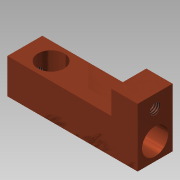
# Autodesk Inventor part: Part26
Saved by Autodesk Inventor 2014 (Build 180170000, 170)
## iProperties
Created: 2015-09-27
Part Number: Part26
Material: Copper
Document SubType Name: Modeling
Designer: Administrator
Density: 1 g/cm^3
Appearance: Copper - Satin
Author: Administrator
Autodesk Inventor part; units mm, degrees
ref_plane "YZ Plane" through (0, 0, 0) normal (1, 0, 0) x (0, 1, 0)
ref_plane "XZ Plane" through (0, 0, 0) normal (0, 1, 0) x (-1, 0, 0)
ref_plane "XY Plane" through (0, 0, 0) normal (0, 0, 1) x (1, 0, 0)
sketch "Sketch1" plane through (0, 0, 0) normal (0, 0, 1) x (1, 0, 0)
  circle A0 centre (0, 0) radius 3 projected
  line L0 (6, -4) -> (-6, -4)
  line L1 (-6, -4) -> (-6, 4)
  line L2 (-6, 4) -> (6, 4)
  line L3 (6, 4) -> (6, -4)
  line L4 (6, -4) -> (-6, 4) construction
  line L5 (-6, -4) -> (6, 4) construction
  line L6 (6, 4) -> (23.8, 4)
  line L7 (23.8, 4) -> (23.8, -4)
  line L8 (23.8, -4) -> (6, -4)
  line L9 (6, -4) -> (6, 4)
  point P0 (0, 0)
  dimension "d0" = 12
  dimension "d1" = 8
  dimension "d2" = 17.8
  constraints: 20 end point, 4 parallel, 2 horizontal, 2 midpoint, 2 perpendicular
  measures "d0" distance of L1.end L2.end
  measures "d1" distance of L0.end L1.end
  measures "d2" distance of L7.end L8.end
extrude "Extrusion1" add sketch "Sketch1" along normal blind 8
sketch "Sketch2" plane through (23.8, -4, 0) normal (1, 0, 0) x (0, 0, -1)
  circle A0 centre (-4, 4) radius 3
  point P0 (0, 4)
  dimension "d5" = 6
  constraints: 1 centre point
  measures "d5" diameter of A0
extrude "Extrusion2" cut sketch "Sketch2" against normal blind 19.8
sketch "Sketch3" plane through (-6, -4, 0) normal (-1, 0, 0) x (0, 0, 1)
  circle A0 centre (4, 4) radius 1.2
  point P0 (0, 4)
  dimension "d8" = 2.4
  constraints: 1 centre point
  measures "d8" diameter of A0
extrude "Extrusion3" cut sketch "Sketch3" against normal blind 4
thread "Thread1" size "M3x0.5" class "6H" standard "ANSI Metric M Profile" full length
sketch "Sketch5" plane through (0, 0, 8) normal (0, 0, 1) x (1, 0, 0)
  line L0 (23.8, 4) -> (-6, 4) projected
  line L1 (-6, -4) -> (23.8, -4) projected
  line L2 (23.8, -4) -> (23.8, 4) projected
  line L3 (17.8, 4) -> (17.8, -4)
  dimension "d20" = 6
  constraints: 2 end point, 2 point on line, 1 perpendicular
  measures "d20" distance between parallel lines of L2 L3
extrude "Extrusion5" add sketch "Sketch5" along normal blind 5.4
sketch "Sketch6" plane through (23.8, -4, 0) normal (1, 0, 0) x (0, 0, -1)
  line L0 (-13.4, 0) -> (-13.4, 8) projected
  circle A0 centre (-10.4, 4) radius 1.2
  point P0 (0, 4)
  dimension "d23" = 2.4
  dimension "d24" = 3
  constraints: 1 centre point
  measures "d23" diameter of A0
  measures "d24" distance from line of L0 A0.centre
extrude "Extrusion6" cut sketch "Sketch6" against normal blind 10
thread "Thread3" size "M3x0.5" class "6H" standard "ANSI Metric M Profile" full length
body "Solid1"
